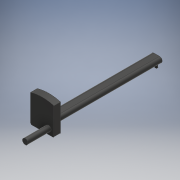
# Autodesk Inventor part: Elektronik
Saved by Autodesk Inventor 2017.3 (Build 213257000, 257)
## iProperties
Created: 2020-01-20
Part Number: Elektronik
Material: Polyethylene, High Density
Document SubType Name: Modeling
Designer: Ole Simmering
Density: 0.952 g/cm^3
Appearance: Smooth - Black
Author: Ole Simmering
Autodesk Inventor part; units mm, degrees
ref_plane "YZ Plane" through (0, 0, 0) normal (1, 0, 0) x (0, 1, 0)
ref_plane "XZ Plane" through (0, 0, 0) normal (0, 1, 0) x (-1, 0, 0)
ref_plane "XY Plane" through (0, 0, 0) normal (0, 0, 1) x (1, 0, 0)
sketch "Sketch1" plane through (0, 0, 0) normal (0, 1, 0) x (-1, 0, 0)
  circle A0 centre (0, 0) radius 75 construction
  arc A1 (21.1092, 71.9681) -> (-21.1092, 71.9681) centre (0, 0) ccw
  line L0 (21.1092, 71.9681) -> (21.1092, 21.9681)
  line L1 (21.1092, 21.9681) -> (-21.1092, 21.9681)
  line L2 (-21.1092, 21.9681) -> (-21.1092, 71.9681)
  line L3 (0, 0) -> (0, 79) construction
  dimension "d0" = 150
  dimension "d1" = 50
  constraints: 8 end point, 2 coincident, 2 perpendicular, 2 point on circle, 1 centre point, 1 parallel, 1 vertical, 4 other
  measures "d1" distance of L0.start L0.end
extrude "Extrusion1" add sketch "Sketch1" along normal blind 12
fillet "Fillet1" radius 2 1 edges at (21.1092, 6, 21.9681)
fillet "Fillet2" radius 2 1 edges at (-21.1092, 6, 21.9681)
sketch "Sketch2" plane through (0, 12, 0) normal (0, 1, 0) x (1, 0, 0)
  line L0 (-10, -33) -> (0, -33)
  line L1 (0, -23) -> (-10, -23)
  arc A0 (-10, -23) -> (-10, -33) centre (-10, -28) ccw
  arc A1 (0, -33) -> (0, -23) centre (0, -28) ccw
  line L2 (19.1092, -21.9681) -> (-19.1092, -21.9681) construction
  line L3 (0, -21.9681) -> (0, -54.4833) construction
  point P0 (0, 0)
  dimension "d6" = 10
  dimension "d7" = 5
  constraints: 6 end point, 4 point on circle, 4 tangent, 2 centre point, 1 midpoint, 1 parallel, 1 point on line, 1 vertical
  measures "d6" distance of A1.centre A0.centre
  measures "d7" radius of A0
extrude "Extrusion2" add sketch "Sketch2" along normal blind 200
sketch "Sketch3" plane through (0, 212, 0) normal (0, 1, 0) x (1, 0, 0)
  line L0 (-12.1019, -31) -> (-10, -31)
  line L1 (-10, -31) -> (-10, -25)
  line L2 (-10, -25) -> (-12.1019, -25)
  line L3 (-12.1019, -25) -> (-12.1019, -31)
  line L4 (-15, -28) -> (5, -28) construction
  circle A0 centre (0, -28) radius 4
  circle A1 centre (-7, -26) radius 2.5
  point P0 (0, 0)
  dimension "d10" = 5
  constraints: 10 end point, 2 centre point, 2 parallel, 1 horizontal, 1 perpendicular, 1 other
  measures "d10" diameter of A1
extrude "Extrusion3" cut sketch "Sketch3" against normal blind 200 contours A0 | A1
sketch "Sketch4" plane through (0, 212, 0) normal (0, 1, 0) x (1, 0, 0)
  line L0 (-15, -28) -> (5, -28) construction
  line L1 (-11, -30) -> (-12.2379, -30)
  line L2 (-12.2379, -30) -> (-12.2379, -26)
  line L3 (-12.2379, -26) -> (-11, -26)
  line L4 (-11, -26) -> (-11, -30)
  point P0 (0, 0)
  constraints: 10 end point, 2 parallel, 1 horizontal, 1 perpendicular, 1 other
extrude "Extrusion4" cut sketch "Sketch4" against normal blind 5
sketch "Sketch5" plane through (0, 212, 0) normal (0, 1, 0) x (1, 0, 0)
  circle A0 centre (-7, -26) radius 2.5 projected
  arc A1 (-10, -26) -> (-4, -26) centre (-7, -26) ccw
  line L0 (-10, -26) -> (-10, -11.0954)
  line L1 (-11, -26) -> (-11, -30) projected
  line L2 (-4, -26) -> (-4, -11.0954)
  line L3 (-10, -11.0954) -> (-4, -11.0954)
  point P0 (0, 0)
  constraints: 6 end point, 2 point on circle, 2 tangent, 1 centre point, 1 coincident, 1 horizontal, 1 parallel, 1 vertical
extrude "Extrusion5" add sketch "Sketch5" along normal blind 2.5 contours A0 | L0 L3 L2 A1
fillet "Fillet3" radius 2 5 edges at (-4, 213.25, 11.0954) (-10, 213.25, 11.0954) (-7, 214.5, 29) (-4, 214.5, 18.5477) (-10, 214.5, 18.5477)
sketch "Sketch6" plane through (0, 0, 0) normal (0, -1, 0) x (1, 0, 0)
  circle A0 centre (11.1092, 31.9681) radius 5
  line L0 (19.1092, 21.9681) -> (-19.1092, 21.9681) projected
  line L1 (21.1092, 71.9681) -> (21.1092, 23.9681) projected
  point P0 (0, 0)
  dimension "d18" = 10
  dimension "d19" = 10
  constraints: 1 centre point
  measures "d18" distance from line of L0 A0.centre
  measures "d19" distance from line of L1 A0.centre
extrude "Extrusion6" add sketch "Sketch6" along normal blind 42
body "Solid1"
